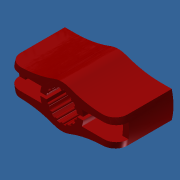
# Autodesk Inventor part: extender-bracket
Saved by Autodesk Inventor 2015 (Build 190159000, 159)
## iProperties
Created: 2019-04-16
Part Number: extender-bracket
Material: Generic
Document SubType Name: Modeling
Designer: gabriel
Density: 1 g/cm^3
Appearance: Default
Author: gabriel
Autodesk Inventor part; units mm, degrees
ref_plane "YZ Plane" through (0, 0, 0) normal (1, 0, 0) x (0, 1, 0)
ref_plane "XZ Plane" through (0, 0, 0) normal (0, 1, 0) x (-1, 0, 0)
ref_plane "XY Plane" through (0, 0, 0) normal (0, 0, 1) x (1, 0, 0)
sketch "Sketch10" plane through (0, 0, 0) normal (0, 0, 1) x (1, 0, 0)
  line L0 (0, 6.985) -> (-9.5327, 6.985)
  line L1 (0, 0) -> (-9.5327, 0)
  line L2 (-18.1754, 0) -> (-27.7081, 0)
  line L3 (-27.7081, 6.985) -> (-18.1754, 6.985)
  arc A0 (-9.5327, 6.985) -> (-18.1754, 6.985) centre (-13.8541, 3.4925) ccw
  arc A1 (-18.1754, 0) -> (-9.5327, 0) centre (-13.8541, 3.4925) ccw
  circle A2 centre (-13.8541, 3.4925) radius 3.9688
  line L4 (-26.4104, 1.5875) -> (-19.0735, 1.5875)
  line L5 (-19.0735, 5.3975) -> (-26.4104, 5.3975)
  line L6 (-8.6346, 1.5875) -> (-1.2978, 1.5875)
  line L7 (-1.2978, 5.3975) -> (-8.6346, 5.3975)
  arc A3 (-19.0735, 5.3975) -> (-19.0735, 1.5875) centre (-13.8541, 3.4925) ccw
  arc A4 (-8.6346, 1.5875) -> (-8.6346, 5.3975) centre (-13.8541, 3.4925) ccw
  arc A5 (-26.4104, 5.3975) -> (-26.4104, 1.5875) centre (-13.8541, 3.4925) ccw
  arc A6 (-27.7081, 6.985) -> (-27.7081, 0) centre (-13.8541, 3.4925) ccw
  arc A7 (-1.2978, 1.5875) -> (-1.2978, 5.3975) centre (-13.8541, 3.4925) ccw
  arc A8 (0, 0) -> (0, 6.985) centre (-13.8541, 3.4925) ccw
  dimension "d59" = 7.9375
  dimension "d152" = 1.5875
  dimension "d153" = 1.5875
  dimension "d158" = 3.81
  dimension "d168" = 12.7
  dimension "d169" = 12.7
  dimension "d170" = 1.5875
  dimension "d172" = 1.5875
  constraints: 16 end point, 16 point on circle, 9 centre point, 8 coincident, 4 horizontal, 3 concentric, 3 equal length, 3 point on line, 2 collinear, 2 parallel
  measures "d59" diameter of A2
  measures "d152" distance between parallel lines of L2 L4
  measures "d153" distance between parallel lines of L3 L5
  measures "d158" distance of L5.end L4.start
  measures "d168" radius of A5
  measures "d169" radius of A7
  measures "d170" radial gap between concentric circles of A6 A5
  measures "d172" radial gap between concentric circles of A0 A2
extrude "Extrusion33" add sketch "Sketch10" along normal blind 14.6844
sketch "Sketch28" plane through (0, 0, 14.6844) normal (0, 0, 1) x (1, 0, 0)
  circle A0 centre (-13.8541, 3.4925) radius 3.9687 projected
  arc A1 (-26.4104, 5.3975) -> (-26.4104, 1.5875) centre (-13.8541, 3.4925) ccw
  arc A2 (-28.014, 5.3975) -> (-28.014, 1.5875) centre (-13.8541, 3.4925) ccw
  arc A3 (-1.2978, 1.5875) -> (-1.2978, 5.3975) centre (-13.8541, 3.4925) ccw
  arc A4 (0.3059, 1.5875) -> (0.3059, 5.3975) centre (-13.8541, 3.4925) ccw
  line L0 (-28.014, 5.3975) -> (-26.4104, 5.3975)
  line L1 (-26.4104, 1.5875) -> (-28.014, 1.5875)
  line L2 (-1.2978, 5.3975) -> (0.3059, 5.3975)
  line L3 (0.3059, 1.5875) -> (-1.2978, 1.5875)
  line L4 (-26.4104, 5.3975) -> (-19.0735, 5.3975) projected
  line L5 (-19.0735, 1.5875) -> (-26.4104, 1.5875) projected
  arc A5 (-26.4104, 5.3975) -> (-26.4104, 1.5875) centre (-13.8541, 3.4925) ccw projected
  arc A6 (-27.7081, 6.985) -> (-27.7081, 0) centre (-13.8541, 3.4925) ccw projected
  arc A7 (-1.2978, 1.5875) -> (-1.2978, 5.3975) centre (-13.8541, 3.4925) ccw projected
  arc A8 (0, 0) -> (0, 6.985) centre (-13.8541, 3.4925) ccw projected
  constraints: 8 end point, 8 point on circle, 4 centre point, 4 coincident, 4 collinear, 4 concentric, 2 horizontal
extrude "Extrusion35" cut sketch "Sketch28" against normal blind 3.175 contours A1 L1 A2 L0 | A3 L2 A4 L3
sketch "Sketch30" plane through (0, 0, 14.6844) normal (0, 0, 1) x (1, 0, 0)
  circle A0 centre (-13.8541, 3.4925) radius 3.9687 projected
  circle A1 centre (-13.8541, 7.4612) radius 0.3969
  circle A2 centre (-15.3728, 7.1591) radius 0.3969
  circle A3 centre (-16.6604, 6.2988) radius 0.3969
  circle A4 centre (-17.5207, 5.0113) radius 0.3969
  circle A5 centre (-17.8228, 3.4925) radius 0.3969
  circle A6 centre (-17.5207, 1.9737) radius 0.3969
  circle A7 centre (-16.6604, 0.6862) radius 0.3969
  circle A8 centre (-15.3728, -0.1741) radius 0.3969
  circle A9 centre (-13.8541, -0.4763) radius 0.3969
  circle A10 centre (-12.3353, -0.1741) radius 0.3969
  circle A11 centre (-11.0477, 0.6862) radius 0.3969
  circle A12 centre (-10.1874, 1.9737) radius 0.3969
  circle A13 centre (-9.8853, 3.4925) radius 0.3969
  circle A14 centre (-10.1874, 5.0113) radius 0.3969
  circle A15 centre (-11.0477, 6.2988) radius 0.3969
  circle A16 centre (-12.3353, 7.1591) radius 0.3969
  point P0 (0, 0)
  dimension "d179" = 0.7937
  dimension "d182" = 360
  constraints: 16 centre point, 2 vertical alignment, 34 other
  measures "d179" diameter of A1
fillet "Fillet6" radius 25.4 4 edges at (-9.5327, 6.985, 7.3422) (-18.1754, 6.985, 7.3422) (-9.5327, 0, 7.3422) (-18.1754, 0, 7.3422)
fillet "Fillet7" radius 3.175 4 edges at (0.1754, 6.1956, 14.6844) (0.1754, 0.7894, 14.6844) (-27.8835, 6.1956, 14.6844) (-27.8835, 0.7894, 14.6844)
extrude "Extrusion41" add sketch "Sketch30" against normal up to surface (14.6844 mm away) contours A0 A13 | A0 A13 | A14 A0 | A0 A14 | A12 A0 | A0 A12 | A15 A0 | A0 A15 | A11 A0 | A0 A11 | A16 A0 | A0 A16 | A10 A0 | A0 A10 | A1 A0 | A0 A1 | A9 A0 | A0 A9 | A2 A0 | A0 A2 | A8 A0 | A0 A8 | A3 A0 | A0 A3 | A7 A0 | A0 A7 | A4 A0 | A0 A4 | A6 A0 | A0 A6 | A5 A0 | A0 A5
sketch "Sketch33" plane through (0, 0, 14.6844) normal (0, 0, 1) x (1, 0, 0)
  line L0 (-19.4103, 3.8894) -> (-8.2978, 3.8894)
  line L1 (-8.2978, 3.8894) -> (-8.2978, 3.0956)
  line L2 (-8.2978, 3.0956) -> (-19.4103, 3.0956)
  line L3 (-19.4103, 3.0956) -> (-19.4103, 3.8894)
  arc A0 (-17.803, 3.0961) -> (-17.803, 3.8889) centre (-17.8228, 3.4925) ccw projected
  arc A1 (-8.6346, 1.5875) -> (-8.6346, 5.3975) centre (-13.8541, 3.4925) ccw projected
  arc A2 (-19.0735, 5.3975) -> (-19.0735, 1.5875) centre (-13.8541, 3.4925) ccw projected
  point P0 (0, 0)
  constraints: 8 end point, 4 tangent, 2 parallel, 1 horizontal, 1 perpendicular
extrude "Extrusion42" cut sketch "Sketch33" against normal through all
body "Solid5"
